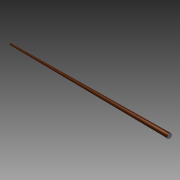
# Autodesk Inventor part: CueStickFull
Saved by Autodesk Inventor 2015 (Build 190159000, 159)
## iProperties
Created: 2017-01-04
Part Number: CueStickFull
Material: Generic
Document SubType Name: Modeling
Designer: Ernest
Density: 1 g/cm^3
Appearance: Default
Author: Ernest
Autodesk Inventor part; units mm, degrees
ref_plane "YZ Plane" through (0, 0, 0) normal (1, 0, 0) x (0, 1, 0)
ref_plane "XZ Plane" through (0, 0, 0) normal (0, 1, 0) x (-1, 0, 0)
ref_plane "XY Plane" through (0, 0, 0) normal (0, 0, 1) x (1, 0, 0)
sketch "Sketch1" plane through (0, 0, 0) normal (0, 0, 1) x (1, 0, 0)
  line L0 (0, 0) -> (1524, 0)
  line L1 (0, 0) -> (0, 7)
  line L2 (0, 0) -> (0, -7)
  line L3 (1524, 0) -> (1524, 22)
  line L4 (1524, 0) -> (1524, -22)
  line L5 (1524, -22) -> (0, -7)
  line L6 (1524, 22) -> (0, 7)
  dimension "d0" = 1524
  dimension "d1" = 7
  dimension "d2" = 7
  dimension "d3" = 22
  dimension "d4" = 22
  constraints: 14 end point, 4 vertical, 1 horizontal
  measures "d0" distance of L0.start L0.end
  measures "d1" distance of L0.start L1.end
  measures "d2" distance of L0.start L2.end
  measures "d3" distance of L0.end L3.end
  measures "d4" distance of L0.end L4.end
revolve "Revolution1" add sketch "Sketch1" angle 360 about axis through (0, 0, 0) along (1, 0, 0) contours L1 L6 L3 L0
body "Solid1"
